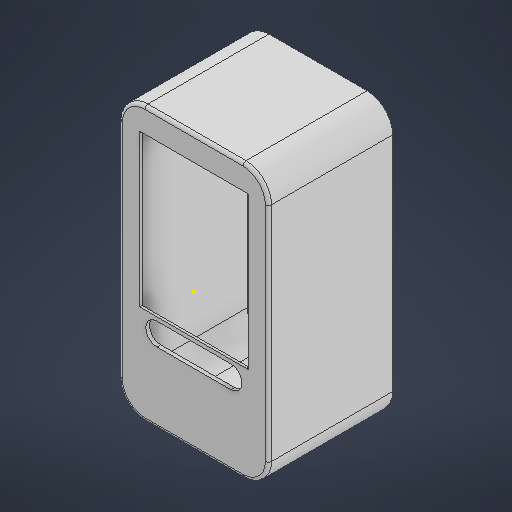
# Autodesk Inventor part: MainBody
Saved by Autodesk Inventor 2026 (Build 300175050, 175E)
## iProperties
Created: 2026-03-28
Part Number: MainBody
Material: Generic
Document SubType Name: Modeling
Designer: tp2105
Density: 1 g/cm^3
Appearance: Default
Author: tp2105
Autodesk Inventor part; units mm, degrees
ref_plane "YZ Plane" through (0, 0, 0) normal (1, 0, 0) x (0, 1, 0)
ref_plane "XZ Plane" through (0, 0, 0) normal (0, 1, 0) x (-1, 0, 0)
ref_plane "XY Plane" through (0, 0, 0) normal (0, 0, 1) x (1, 0, 0)
sketch "Sketch1" plane through (0, 0, 0) normal (0, 0, 1) x (1, 0, 0)
  line L0 (0, 0) -> (100, 0) construction
  line L1 (-30, -55) -> (30, -55)
  line L2 (30, -55) -> (30, 55)
  line L3 (30, 55) -> (-30, 55)
  line L4 (-30, 55) -> (-30, -55)
  line L5 (-30, -55) -> (30, 55) construction
  line L6 (30, -55) -> (-30, 55) construction
  dimension "d5" = 60
  dimension "d6" = 110
  constraints: 14 end point, 2 horizontal, 2 midpoint, 2 parallel, 1 perpendicular
  measures "d5" distance of L3.end L2.end
  measures "d6" distance of L2.end L1.end
extrude "Extrusion1" add sketch "Sketch1" along normal mid plane 50
fillet "Fillet1" radius 10.25 4 edges at (30, 55, 0) (-30, 55, 0) (30, -55, 0) (-30, -55, 0)
fillet "Fillet2" radius 1.25 8 edges at (-26.9978, 51.9978, 25) (-30, 0, 25) (-26.9978, -51.9978, 25) (0, -55, 25) (26.9978, -51.9978, 25) (30, 0, 25) (26.9978, 51.9978, 25) (0, 55, 25)
sketch "Sketch3" plane through (0, 0, 25) normal (0, 0, 1) x (1, 0, 0)
  line L0 (-21.36, 44.6065) -> (21.36, 44.6065)
  line L1 (21.36, 44.6065) -> (21.36, -15.6535)
  line L2 (21.36, -15.6535) -> (-21.36, -15.6535)
  line L3 (-21.36, -15.6535) -> (-21.36, 44.6065)
  line L4 (-21.36, 44.6065) -> (21.36, -15.6535) construction
  line L5 (21.36, 44.6065) -> (-21.36, -15.6535) construction
  point P0 (0, 0)
  point P1 (0, 14.4765)
  dimension "d21" = 42.72
  dimension "d22" = 60.26
  constraints: 12 end point, 2 midpoint, 2 parallel, 1 horizontal, 1 perpendicular
  measures "d21" distance of L1.end L2.end
  measures "d22" distance of L0.end L1.end
extrude "Extrusion3" cut sketch "Sketch3" against normal blind 0.5
shell "Shell2" thickness 1.5 removed faces 2 at (7.12, 4.4332, 24.5) at (-10, 14.9167, -25)
fillet "Fillet4" radius 0.5 4 edges at (-21.36, 14.4765, 25) (0, 44.6065, 25) (21.36, 14.4765, 25) (0, -15.6535, 25)
sketch "Sketch4" plane through (0, 0, 25) normal (0, 0, 1) x (1, 0, 0)
  line L0 (-21.86, -16.1535) -> (21.86, -16.1535) projected
  line L1 (21.86, -16.1535) -> (2.86, -16.1535)
  line L2 (21.86, -16.1535) -> (15.86, -16.1535)
  circle A0 centre (10.86, -22.1535) radius 4
  circle A1 centre (-6.64, -22.1535) radius 2
  line L3 (21.36, -15.6535) -> (-21.36, -15.6535) projected
  line L4 (21.36, -15.6535) -> (14.36, -15.6535)
  circle A2 centre (-6.64, -22.1535) radius 3
  line L5 (-14.86, -22.1535) -> (14.86, -22.1535) construction
  line L6 (-14.86, -26.6535) -> (14.86, -26.6535)
  line L7 (14.86, -17.6535) -> (-14.86, -17.6535)
  arc A3 (-14.86, -17.6535) -> (-14.86, -26.6535) centre (-14.86, -22.1535) ccw
  arc A4 (14.86, -26.6535) -> (14.86, -17.6535) centre (14.86, -22.1535) ccw
  point P0 (0, 0)
  point P1 (0, -22.1535)
  dimension "d33" = 4
  dimension "d35" = 6
  dimension "d36" = 9
  constraints: 14 end point, 4 centre point, 4 point on circle, 4 tangent, 3 point on line, 1 coincident, 1 horizontal, 1 horizontal alignment, 1 midpoint, 1 parallel, 2 other
  measures "d33" diameter of A1
  measures "d35" diameter of A2
  measures "d36" diameter of A4
extrude "Extrusion4" cut sketch "Sketch4" against normal blind 4 contours A0 | A1 | A2 | A3 L7 A4 L6
sketch "Sketch5" plane through (0, 0, 25) normal (0, 0, 1) x (1, 0, 0)
  point P0 (0, 0)
body "Solid1"
